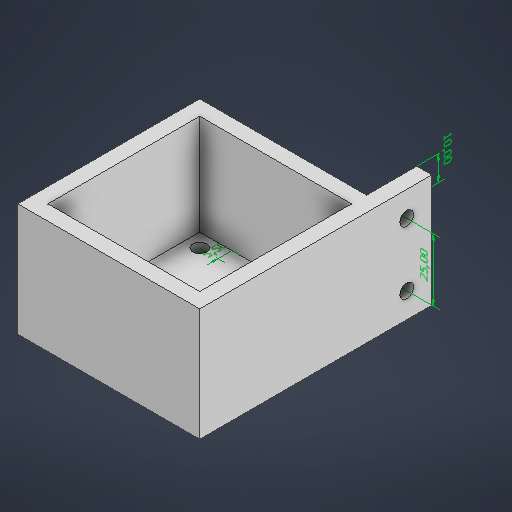
# Autodesk Inventor part: soporte motor
Saved by Autodesk Inventor 2026.1 (Build 301233020, 233B)
## iProperties
Created: 2025-11-23
Part Number: soporte motor
Material: Generic
Document SubType Name: Modeling
Designer: Tito Luyo Murata
Density: 1 g/cm^3
Appearance: Default
Author: Tito Luyo Murata
Autodesk Inventor part; units mm, degrees
ref_plane "YZ Plane" through (0, 0, 0) normal (1, 0, 0) x (0, 1, 0)
ref_plane "XZ Plane" through (0, 0, 0) normal (0, 1, 0) x (-1, 0, 0)
ref_plane "XY Plane" through (0, 0, 0) normal (0, 0, 1) x (1, 0, 0)
sketch "Sketch1" plane through (0, 0, 0) normal (0, 1, 0) x (-1, 0, 0)
  line L0 (0, 0) -> (60.5, 0)
  line L1 (60.5, 0) -> (60.5, -60.5)
  line L2 (60.5, -60.5) -> (0, -60.5)
  line L3 (0, -60.5) -> (0, 0)
  line L4 (-6, -66.5) -> (66.5, -66.5)
  line L5 (66.5, -66.5) -> (66.5, 6)
  line L6 (66.5, 6) -> (-6, 6)
  line L7 (-6, 6) -> (-6, -66.5)
  dimension "d0" = 60.5
  dimension "d1" = 60.5
  dimension "d2" = 6
  constraints: 16 end point, 4 parallel, 2 perpendicular, 1 horizontal, 3 other
  measures "d0" distance of L1.end L2.end
  measures "d1" distance of L0.end L1.end
  measures "d2" distance between parallel lines of L2 L4
extrude "Extrusion1" add sketch "Sketch1" along normal blind 40
sketch "Sketch2" plane through (0, 0, 0) normal (0, -1, 0) x (1, 0, 0)
  line L0 (-66.5, -60.5) -> (-66.5, 6)
  line L1 (-66.5, 6) -> (6, 6)
  line L2 (6, 6) -> (6, -66.5)
  line L3 (6, -66.5) -> (-66.5, -66.5)
  line L4 (-66.5, -66.5) -> (-66.5, 6)
  point P0 (0, 0)
  point P1 (-63.5, -63.5)
  dimension "d5" = 72.5
  dimension "d6" = 72.5
  dimension "d62" = 6
  dimension "d63" = 6
  constraints: 10 end point, 2 parallel, 1 horizontal, 1 perpendicular
  measures "d5" distance of L2.end L3.end
  measures "d6" distance of L1.end L2.end
  measures "d62" distance from line of point (0, 0) L1
  measures "d63" distance from line of point (0, 0) L2
extrude "Extrusion2" add sketch "Sketch2" along normal blind 5
sketch "Sketch3" plane through (0, -5, 0) normal (0, -1, 0) x (1, 0, 0)
  line L0 (20, -30.25) -> (-80, -30.25) construction
  line L1 (-30.25, 20) -> (-30.25, -80) construction
  circle A0 centre (-55, -5.5) radius 2.8
  circle A1 centre (-5.5, -5.5) radius 2.8
  circle A2 centre (-55, -55) radius 2.8
  circle A3 centre (-5.5, -55) radius 2.8
  point P0 (0, 0)
  dimension "d9" = 100
  dimension "d10" = 30.25
  dimension "d11" = 100
  dimension "d12" = 30.25
  dimension "d13" = 24.75
  dimension "d14" = 24.75
  dimension "d15" = 5.6
  dimension "d18" = 49.5
  dimension "d21" = 49.5
  constraints: 4 centre point, 4 end point, 2 horizontal, 2 vertical, 6 other
  measures "d9" distance of L0.start L0.end
  measures "d10" distance from line of point (0, 0) L0
  measures "d11" distance of L1.start L1.end
  measures "d12" distance from line of point (0, 0) L1
  measures "d13" distance from line of L1 A0.centre
  measures "d14" distance from line of L0 A0.centre
  measures "d15" diameter of A0
  measures "d18" distance of A0.centre A1.centre
  measures "d21" distance of A0.centre A2.centre
extrude "Extrusion3" cut sketch "Sketch3" against normal blind 5
sketch "Sketch4" plane through (0, 0, 0) normal (0, 1, 0) x (1, 0, 0)
  line L0 (20, 30.25) -> (-80, 30.25) construction
  line L1 (0, 0) -> (-60.5, 0) construction
  line L2 (-30.25, -20) -> (-30.25, 80) construction
  line L3 (0, 60.5) -> (0, 0) construction
  circle A0 centre (-30.25, 20.25) radius 12.5
  dimension "d26" = 100
  dimension "d27" = 30.25
  dimension "d28" = 100
  dimension "d29" = 30.25
  dimension "d30" = 25
  dimension "d31" = 10
  constraints: 4 end point, 1 centre point, 1 horizontal, 1 point on line, 1 vertical
  measures "d26" distance of L0.start L0.end
  measures "d27" distance between parallel lines of L1 L0
  measures "d28" distance of L2.start L2.end
  measures "d29" distance between parallel lines of L3 L2
  measures "d30" diameter of A0
  measures "d31" distance from line of L0 A0.centre
extrude "Extrusion4" cut sketch "Sketch4" against normal blind 3.3
sketch "Sketch5" plane through (-30.25, -3.3, -20.25) normal (0, 1, 0) x (1, 0, 0)
  circle A0 centre (0, 0) radius 4.5
  point P0 (30.25, -20.25)
  dimension "d34" = 9
  constraints: 1 centre point
  measures "d34" diameter of A0
extrude "Extrusion5" cut sketch "Sketch5" against normal blind 2
sketch "Sketch8" plane through (6, 40, -66.5) normal (0, 0, -1) x (-1, 0, 0)
  line L0 (0, 0) -> (72.5, 0) projected
  line L1 (0, -45) -> (72.5, -45) projected
  line L2 (0, 0) -> (6, 0)
  line L3 (6, 0) -> (6, -45)
  line L4 (6, -45) -> (0, -45)
  line L5 (0, -45) -> (0, 0)
  point P0 (6, -40)
  dimension "d64" = 6
  constraints: 8 end point, 2 parallel, 1 horizontal, 1 perpendicular, 1 point on line
  measures "d64" distance of L3.end L4.end
extrude "Extrusion8" add sketch "Sketch8" along normal blind 20
sketch "Sketch9" plane through (0, -5, -66.5) normal (-1, 0, 0) x (0, 0, 1)
  circle A0 centre (-10, 10) radius 2.75
  line L0 (-20, 0) -> (-20, 45) projected
  line L1 (0, 0) -> (-20, 0) projected
  circle A1 centre (-10, 35) radius 2.75
  line L2 (0, 45) -> (-20, 45) projected
  point P0 (66.5, 5)
  dimension "d67" = 5.5
  dimension "d68" = 10
  dimension "d69" = 10
  dimension "d70" = 5.5
  dimension "d71" = 10
  dimension "d72" = 10
  constraints: 2 centre point
  measures "d67" diameter of A0
  measures "d68" distance from line of A0.centre L0
  measures "d69" distance from line of L1 A0.centre
  measures "d70" diameter of A1
  measures "d71" distance from line of L2 A1.centre
  measures "d72" distance from line of A1.centre L0
extrude "Extrusion9" cut sketch "Sketch9" against normal blind 6
body "Solid1"
